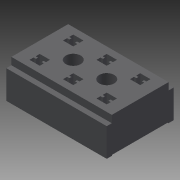
# Autodesk Inventor part: CLT-103-01-F-D_socket
Saved by Autodesk Inventor 2014 SP2 (Build 180246200, 246)
## iProperties
Created: 2019-03-13
Part Number: CLT-103-01-F-D_socket
Material: Generic
Catalog Web Link: www.cadenas.de
Description: CLT Series Socket-CLT Series - (2,00 mm) .0787'' Low Profile Dual Wipe Socket
Vendor: SAMTEC
Document SubType Name: Modeling
Designer: psadmin
Manufacturer: SAMTEC
Mass: 0.0404172 g
Surface Area: 1.33398 cm^2
Volume: 0.0404172 cm^3
Density: 1 g/cm^3
Appearance: PSOLRGB-127-127-127
Category: PARTsolutions
Company: SAMTEC
Title: CLT-103-01-F-D_socket
Author: Cadenas PARTsolutions
Comments: CLT Series - (2,00 mm) .0787'' Low Profile Dual Wipe Socket
PSOL_IDENT_0: {$CADENAS_DATA\23d-libs\samtec\modelling\clt\parts\clt_socket.prj},228 {VTYP=3D},{NB=CLT-103-01-F-D_
PSOL_IDENT_1: socket},{LINA=CLT-103-01-F-D_socket},{NN=CLT Series Socket},{DATE=01.08.2018 08:15:54},{GEOMDATE=14.
PSOL_IDENT_2: 04.2016 10:51:00},{VERSION=},{LINEID=10},{WBVAR=POS,LS,PLOPT,AOPT,TROPT,BEOPT,PPOPT},{WBNUMERIC=}  {
PSOL_IDENT_3: NB=CLT-103-01-F-D_socket},{LINA=CLT-103-01-F-D_socket},{KT=DUMMY},{PN=CLT-103-01-F-D},{SERIES=CLT},{
PSOL_IDENT_4: POS=03},{POSN=3},{POSALG=  '02' , '-02' , '03' , '-03' , '04' , '-04' , '05' , '-05' , '06' , '-06'
PSOL_IDENT_5: , '07' , '-07' , '08' , '-08' , '09' , '-09' , '10' , '-10' , '11' , '-11' , '12' , '-12' , '13' , '
PSOL_IDENT_6: -13' , '14' , '-14' , '15' , '-15' , '16' , '-16' , '17' , '-17' , '18' , '-18' , '19' , '-19' , '20'
PSOL_IDENT_7: , '-20' , '21' , '-21' , '22' , '-22' , '23' , '-23' , '24' , '-24' , '25' , '-25' , '26' , '-26' ,
PSOL_IDENT_8: '27' , '-27' , '28' , '-28' , '29' , '-29' , '30' , '-30' , '31' , '-31' , '32' , '-32' , '33' , '-
PSOL_IDENT_9: 33' , '34' , '-34' , '35' , '-35' , '36' , '-36' , '37' , '-37' , '38' , '-38' , '39' , '-39' , '40'
PSOL_IDENT_10: , '-40' , '41' , '-41' , '42' , '-42' , '43' , '-43' , '44' , '-44' , '45' , '-45' , '46' , '-46' ,
PSOL_IDENT_11: '47' , '-47' , '48' , '-48' , '49' , '-49' , '50' , '-50'  },{POSPN=03},{LS=01},{PLOPT=F},{PLOPTALG=
PSOL_IDENT_12: 'G','-G = Gold, 10 Au / 50 Ni min on Contact, 3 Au / 50 Ni min on Tail.','S','-S = Selective, 30 Au
PSOL_IDENT_13: / 50 Ni min on Contact, Matte Tin Tail.','F','-F = Flash Selective, 3 Au / 50 Ni min on Contact, Ma
PSOL_IDENT_14: tte Tin Tail.','SM','-SM = Selective, 30 Au / 50 Ni min on Contact, Matte Tin Tail.','FM','-FM = Fla
PSOL_IDENT_15: sh Selective, 3 Au / 50 Ni min on Contact, Matte Tin Tail.','L','-L = Light Selective, 10 Au / 50 Ni
PSOL_IDENT_16: min on Contact, Matte Tin Tail.','LM','-LM = Light Selective, 100 Au / 50 Ni min on Contact, Matte
PSOL_IDENT_17: Tin Tail.' },{ROW=Double Row},{AOPT=},{AOPTALG= '','Not Available' },{AOPTPN=},{TROPT=},{TROPTALG= ''
PSOL_IDENT_18: ,'Not Available' },{TROPTPN=},{BEOPT=},{BEOPTALG= '','Not Available' },{BEOPTPN=},{PPOPT=},{PPOPTALG=
PSOL_IDENT_19: '','Not Available' },{PPOPTPN=},{A=0.085},{W=0.23622}
NN: CLT Series Socket
NT: CLT Series - (2,00 mm) .0787'' Low Profile Dual Wipe Socket
NB: CLT-103-01-F-D_socket
NBSYN: $PN._socket
LINA: CLT-103-01-F-D_socket
PN: CLT-103-01-F-D
SERIES: CLT
POS: -03
LS: -01
PLOPT: -F = Flash Selective, 3 Au / 50 Ni min on Contact, Matte Tin Tail.
ROW: Double Row
AOPT: Not Available
TROPT: Not Available
BEOPT: Not Available
PPOPT: Not Available
A: 0.085
SUPPLIER: SAMTEC
ARTICLENO: CLT-103-01-F-D_socket
BOMINFO: CLT-103-01-F-D_socket
CREATOR: CADENAS GmbH
Autodesk Inventor part; units mm, degrees
sketch "Sketch_1" plane through (0, 0, 0) normal (0, 1, 0) x (-1, 0, 0)
  line L0 (0, -2.0003) -> (0, 2.0003)
  line L1 (0, 2.0003) -> (-6, 2.0003)
  line L2 (-6, 2.0003) -> (-6, -2.0003)
  line L3 (-6, -2.0003) -> (0, -2.0003)
  line L4 (-4.6952, 1.0635) -> (-4.6952, 1.3048)
  line L5 (-4.6952, 1.3048) -> (-5.3048, 1.3048)
  line L6 (-5.3048, 1.3048) -> (-5.3048, 1.0635)
  line L7 (-5.3048, 1.0635) -> (-5.1651, 1.0635)
  line L8 (-5.1651, 1.0635) -> (-5.1651, 0.9365)
  line L9 (-5.1651, 0.9365) -> (-5.3048, 0.9365)
  line L10 (-5.3048, 0.9365) -> (-5.3048, 0.6952)
  line L11 (-5.3048, 0.6952) -> (-4.6952, 0.6952)
  line L12 (-4.6952, 0.6952) -> (-4.6952, 0.9365)
  line L13 (-4.6952, 0.9365) -> (-4.8349, 0.9365)
  line L14 (-4.8349, 0.9365) -> (-4.8349, 1.0635)
  line L15 (-4.8349, 1.0635) -> (-4.6952, 1.0635)
  line L16 (-4.6952, -0.9365) -> (-4.6952, -0.6952)
  line L17 (-4.6952, -0.6952) -> (-5.3048, -0.6952)
  line L18 (-5.3048, -0.6952) -> (-5.3048, -0.9365)
  line L19 (-5.3048, -0.9365) -> (-5.1651, -0.9365)
  line L20 (-5.1651, -0.9365) -> (-5.1651, -1.0635)
  line L21 (-5.1651, -1.0635) -> (-5.3048, -1.0635)
  line L22 (-5.3048, -1.0635) -> (-5.3048, -1.3048)
  line L23 (-5.3048, -1.3048) -> (-4.6952, -1.3048)
  line L24 (-4.6952, -1.3048) -> (-4.6952, -1.0635)
  line L25 (-4.6952, -1.0635) -> (-4.8349, -1.0635)
  line L26 (-4.8349, -1.0635) -> (-4.8349, -0.9365)
  line L27 (-4.8349, -0.9365) -> (-4.6952, -0.9365)
  line L28 (-2.6952, 1.0635) -> (-2.6952, 1.3048)
  line L29 (-2.6952, 1.3048) -> (-3.3048, 1.3048)
  line L30 (-3.3048, 1.3048) -> (-3.3048, 1.0635)
  line L31 (-3.3048, 1.0635) -> (-3.1651, 1.0635)
  line L32 (-3.1651, 1.0635) -> (-3.1651, 0.9365)
  line L33 (-3.1651, 0.9365) -> (-3.3048, 0.9365)
  line L34 (-3.3048, 0.9365) -> (-3.3048, 0.6952)
  line L35 (-3.3048, 0.6952) -> (-2.6952, 0.6952)
  line L36 (-2.6952, 0.6952) -> (-2.6952, 0.9365)
  line L37 (-2.6952, 0.9365) -> (-2.8349, 0.9365)
  line L38 (-2.8349, 0.9365) -> (-2.8349, 1.0635)
  line L39 (-2.8349, 1.0635) -> (-2.6952, 1.0635)
  line L40 (-2.6952, -0.9365) -> (-2.6952, -0.6952)
  line L41 (-2.6952, -0.6952) -> (-3.3048, -0.6952)
  line L42 (-3.3048, -0.6952) -> (-3.3048, -0.9365)
  line L43 (-3.3048, -0.9365) -> (-3.1651, -0.9365)
  line L44 (-3.1651, -0.9365) -> (-3.1651, -1.0635)
  line L45 (-3.1651, -1.0635) -> (-3.3048, -1.0635)
  line L46 (-3.3048, -1.0635) -> (-3.3048, -1.3048)
  line L47 (-3.3048, -1.3048) -> (-2.6952, -1.3048)
  line L48 (-2.6952, -1.3048) -> (-2.6952, -1.0635)
  line L49 (-2.6952, -1.0635) -> (-2.8349, -1.0635)
  line L50 (-2.8349, -1.0635) -> (-2.8349, -0.9365)
  line L51 (-2.8349, -0.9365) -> (-2.6952, -0.9365)
  line L52 (-0.6952, 1.0635) -> (-0.6952, 1.3048)
  line L53 (-0.6952, 1.3048) -> (-1.3048, 1.3048)
  line L54 (-1.3048, 1.3048) -> (-1.3048, 1.0635)
  line L55 (-1.3048, 1.0635) -> (-1.1651, 1.0635)
  line L56 (-1.1651, 1.0635) -> (-1.1651, 0.9365)
  line L57 (-1.1651, 0.9365) -> (-1.3048, 0.9365)
  line L58 (-1.3048, 0.9365) -> (-1.3048, 0.6952)
  line L59 (-1.3048, 0.6952) -> (-0.6952, 0.6952)
  line L60 (-0.6952, 0.6952) -> (-0.6952, 0.9365)
  line L61 (-0.6952, 0.9365) -> (-0.8349, 0.9365)
  line L62 (-0.8349, 0.9365) -> (-0.8349, 1.0635)
  line L63 (-0.8349, 1.0635) -> (-0.6952, 1.0635)
  line L64 (-0.6952, -0.9365) -> (-0.6952, -0.6952)
  line L65 (-0.6952, -0.6952) -> (-1.3048, -0.6952)
  line L66 (-1.3048, -0.6952) -> (-1.3048, -0.9365)
  line L67 (-1.3048, -0.9365) -> (-1.1651, -0.9365)
  line L68 (-1.1651, -0.9365) -> (-1.1651, -1.0635)
  line L69 (-1.1651, -1.0635) -> (-1.3048, -1.0635)
  line L70 (-1.3048, -1.0635) -> (-1.3048, -1.3048)
  line L71 (-1.3048, -1.3048) -> (-0.6952, -1.3048)
  line L72 (-0.6952, -1.3048) -> (-0.6952, -1.0635)
  line L73 (-0.6952, -1.0635) -> (-0.8349, -1.0635)
  line L74 (-0.8349, -1.0635) -> (-0.8349, -0.9365)
  line L75 (-0.8349, -0.9365) -> (-0.6952, -0.9365)
  constraints: 152 end point
extrude "Extrusion1" add sketch "Sketch_1" along normal blind 2.1209
sketch "Sketch_7" plane through (0, 0, 0) normal (1, 0, 0) x (0, 1, 0)
  line L0 (0.0508, 1.6853) -> (0, 1.6853)
  line L1 (0, 1.6853) -> (0, -1.6853)
  line L2 (0, -1.6853) -> (0.0508, -1.6853)
  line L3 (0.0508, -1.6853) -> (0.0508, 1.6853)
  constraints: 8 end point
extrude "Extrusion2" cut sketch "Sketch_7" along normal blind 6
sketch "Sketch_8" plane through (0, 0, 0) normal (1, 0, 0) x (0, 1, 0)
  line L0 (2.9591, 2.9655) -> (1.6891, 2.9655)
  line L1 (1.6891, 2.9655) -> (1.6891, 1.6955)
  line L2 (1.6891, 1.6955) -> (2.1209, 1.6955)
  line L3 (2.1209, 1.6955) -> (2.1209, -1.6955)
  line L4 (2.1209, -1.6955) -> (1.6891, -1.6955)
  line L5 (1.6891, -1.6955) -> (1.6891, -2.9655)
  line L6 (1.6891, -2.9655) -> (2.9591, -2.9655)
  line L7 (2.9591, -2.9655) -> (2.9591, 2.9655)
  constraints: 16 end point
extrude "Extrusion3" cut sketch "Sketch_8" along normal blind 6
sketch "Sketch4" plane through (0, 2.1209, 0) normal (0, 1, 0) x (1, 0, 0)
  point P0 (2, 0)
hole "Hole1" at (2, 2.1209, 0) direction (0, -1, 0) diameter 0.889 depth 1.143
pattern_linear "Rectangular Pattern1" count 2 spacing 2 along (1, 0, 0) of "Hole1"
sketch "Sketch_12" plane through (0, 0, 0) normal (0, 1, 0) x (-1, 0, 0)
  line L0 (-0.4285, 0.6032) -> (-0.4285, 1.5938)
  line L1 (-0.4285, 1.5938) -> (-1.5715, 1.5938)
  line L2 (-1.5715, 1.5938) -> (-1.5715, 0.6032)
  line L3 (-1.5715, 0.6032) -> (-0.4285, 0.6032)
  constraints: 8 end point
extrude "Extrusion4" cut sketch "Sketch_12" along normal blind 0.5302
pattern_linear "Rectangular Pattern2" count 3 spacing 2 along (1, 0, 0) count 2 spacing 2.1971 along (0, 0, -1) of "Extrusion4"
ref_plane "socket_XY" through (3, 0, 0) normal (0, 1, 0) x (1, 0, 0)
ref_plane "socket_YZ" through (3, 0, 0) normal (1, 0, 0) x (0, 0, -1)
ref_plane "socket_ZX" through (3, 0, 0) normal (0, 0, -1) x (0, 1, 0)
ref_plane "to_alignment_pin_1_XY" through (2, 0.0508, 0) normal (0, 1, 0) x (1, 0, 0)
ref_plane "to_alignment_pin_1_YZ" through (2, 0.0508, 0) normal (1, 0, 0) x (0, 0, -1)
ref_plane "to_alignment_pin_1_ZX" through (2, 0.0508, 0) normal (0, 0, -1) x (0, 1, 0)
ref_plane "to_alignment_pin_2_XY" through (4, 0.0508, 0) normal (0, 1, 0) x (1, 0, 0)
ref_plane "to_alignment_pin_2_YZ" through (4, 0.0508, 0) normal (1, 0, 0) x (0, 0, -1)
ref_plane "to_alignment_pin_2_ZX" through (4, 0.0508, 0) normal (0, 0, -1) x (0, 1, 0)
ref_plane "to_pick_and_place_pad_XY" through (3, 2.1209, 0) normal (0, 1, 0) x (1, 0, 0)
ref_plane "to_pick_and_place_pad_YZ" through (3, 2.1209, 0) normal (1, 0, 0) x (0, 0, -1)
ref_plane "to_pick_and_place_pad_ZX" through (3, 2.1209, 0) normal (0, 0, -1) x (0, 1, 0)
ref_plane "to_polyimide_film_pad_XY" through (3, 2.1209, 0) normal (0, 1, 0) x (1, 0, 0)
ref_plane "to_polyimide_film_pad_YZ" through (3, 2.1209, 0) normal (1, 0, 0) x (0, 0, -1)
ref_plane "to_polyimide_film_pad_ZX" through (3, 2.1209, 0) normal (0, 0, -1) x (0, 1, 0)
body "Solid1"
